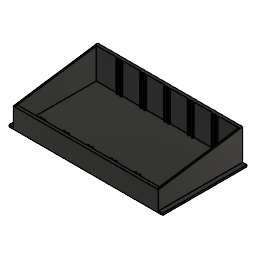
bin (Autodesk Fusion 360 design; units mm, degrees)
part number: 2026-08-18-20-33-51-830
Autodesk Fusion 360 part; units mm, degrees
sketch "Sketch1" plane through (0, 0, 0) normal (0, 0, 1) x (1, 0, 0)
  line L0 (-6, 0) -> (207, 0)
  line L1 (207, 0) -> (207, 117)
  line L2 (207, 117) -> (-6, 117)
  line L3 (-6, 117) -> (-6, 0)
extrude "Extrude1" add sketch "Sketch1" along normal blind 2.4 makes body 1
sketch "Sketch2" plane through (0, 0, 0) normal (0, 0, 1) x (1, 0, 0)
  line L0 (0, 0) -> (201, 0)
  line L1 (201, 0) -> (201, 4)
  line L2 (201, 4) -> (0, 4)
  line L3 (0, 4) -> (0, 0)
extrude "Extrude2" add sketch "Sketch2" along normal blind 28 separate body makes body 2
sketch "Sketch3" plane through (0, 0, 0) normal (0, 0, 1) x (1, 0, 0)
  line L0 (0, 113) -> (201, 113)
  line L1 (201, 113) -> (201, 117)
  line L2 (201, 117) -> (0, 117)
  line L3 (0, 117) -> (0, 113)
extrude "Extrude3" add sketch "Sketch3" along normal blind 45 separate body makes body 3
sketch "Sketch4" plane through (0, 0, 0) normal (1, 0, 0) x (0, 0, -1)
  line L0 (0, 0) -> (0, 117)
  line L1 (0, 117) -> (-45, 117)
  line L2 (-45, 117) -> (-28, 0)
  line L3 (-28, 0) -> (0, 0)
extrude "Extrude4" add sketch "Sketch4" along normal blind 2 separate body makes body 4
sketch "Sketch5" plane through (0, 0, 0) normal (1, 0, 0) x (0, 0, -1)
  line L0 (0, 0) -> (0, 117)
  line L1 (0, 117) -> (-45, 117)
  line L2 (-45, 117) -> (-28, 0)
  line L3 (-28, 0) -> (0, 0)
extrude "Extrude5" add sketch "Sketch5" along normal blind 2 from surface at 199 separate body makes body 5
sketch "Sketch6" plane through (0, 0, 0) normal (0, 0, 1) x (1, 0, 0)
  line L0 (31.4, 4) -> (33.4, 4)
  line L1 (33.4, 4) -> (33.4, 6)
  line L2 (33.4, 6) -> (31.4, 6)
  line L3 (31.4, 6) -> (31.4, 4)
extrude "Extrude6" add sketch "Sketch6" along normal blind 25.6 from surface at 2.4 separate body makes body 6
sketch "Sketch7" plane through (0, 0, 0) normal (0, 0, 1) x (1, 0, 0)
  line L0 (31.4, 111) -> (33.4, 111)
  line L1 (33.4, 111) -> (33.4, 113)
  line L2 (33.4, 113) -> (31.4, 113)
  line L3 (31.4, 113) -> (31.4, 111)
extrude "Extrude7" add sketch "Sketch7" along normal blind 42.6 from surface at 2.4 separate body makes body 7
sketch "Sketch8" plane through (0, 0, 0) normal (0, 0, 1) x (1, 0, 0)
  line L0 (36.6, 4) -> (38.6, 4)
  line L1 (38.6, 4) -> (38.6, 6)
  line L2 (38.6, 6) -> (36.6, 6)
  line L3 (36.6, 6) -> (36.6, 4)
extrude "Extrude8" add sketch "Sketch8" along normal blind 25.6 from surface at 2.4 separate body makes body 8
sketch "Sketch9" plane through (0, 0, 0) normal (0, 0, 1) x (1, 0, 0)
  line L0 (36.6, 111) -> (38.6, 111)
  line L1 (38.6, 111) -> (38.6, 113)
  line L2 (38.6, 113) -> (36.6, 113)
  line L3 (36.6, 113) -> (36.6, 111)
extrude "Extrude9" add sketch "Sketch9" along normal blind 42.6 from surface at 2.4 separate body makes body 9
sketch "Sketch10" plane through (0, 0, 0) normal (0, 0, 1) x (1, 0, 0)
  line L0 (64.4, 4) -> (66.4, 4)
  line L1 (66.4, 4) -> (66.4, 6)
  line L2 (66.4, 6) -> (64.4, 6)
  line L3 (64.4, 6) -> (64.4, 4)
extrude "Extrude10" add sketch "Sketch10" along normal blind 25.6 from surface at 2.4 separate body makes body 10
sketch "Sketch11" plane through (0, 0, 0) normal (0, 0, 1) x (1, 0, 0)
  line L0 (64.4, 111) -> (66.4, 111)
  line L1 (66.4, 111) -> (66.4, 113)
  line L2 (66.4, 113) -> (64.4, 113)
  line L3 (64.4, 113) -> (64.4, 111)
extrude "Extrude11" add sketch "Sketch11" along normal blind 42.6 from surface at 2.4 separate body makes body 11
sketch "Sketch12" plane through (0, 0, 0) normal (0, 0, 1) x (1, 0, 0)
  line L0 (69.6, 4) -> (71.6, 4)
  line L1 (71.6, 4) -> (71.6, 6)
  line L2 (71.6, 6) -> (69.6, 6)
  line L3 (69.6, 6) -> (69.6, 4)
extrude "Extrude12" add sketch "Sketch12" along normal blind 25.6 from surface at 2.4 separate body makes body 12
sketch "Sketch13" plane through (0, 0, 0) normal (0, 0, 1) x (1, 0, 0)
  line L0 (69.6, 111) -> (71.6, 111)
  line L1 (71.6, 111) -> (71.6, 113)
  line L2 (71.6, 113) -> (69.6, 113)
  line L3 (69.6, 113) -> (69.6, 111)
extrude "Extrude13" add sketch "Sketch13" along normal blind 42.6 from surface at 2.4 separate body makes body 13
sketch "Sketch14" plane through (0, 0, 0) normal (0, 0, 1) x (1, 0, 0)
  line L0 (97.4, 4) -> (99.4, 4)
  line L1 (99.4, 4) -> (99.4, 6)
  line L2 (99.4, 6) -> (97.4, 6)
  line L3 (97.4, 6) -> (97.4, 4)
extrude "Extrude14" add sketch "Sketch14" along normal blind 25.6 from surface at 2.4 separate body makes body 14
sketch "Sketch15" plane through (0, 0, 0) normal (0, 0, 1) x (1, 0, 0)
  line L0 (97.4, 111) -> (99.4, 111)
  line L1 (99.4, 111) -> (99.4, 113)
  line L2 (99.4, 113) -> (97.4, 113)
  line L3 (97.4, 113) -> (97.4, 111)
extrude "Extrude15" add sketch "Sketch15" along normal blind 42.6 from surface at 2.4 separate body makes body 15
sketch "Sketch16" plane through (0, 0, 0) normal (0, 0, 1) x (1, 0, 0)
  line L0 (102.6, 4) -> (104.6, 4)
  line L1 (104.6, 4) -> (104.6, 6)
  line L2 (104.6, 6) -> (102.6, 6)
  line L3 (102.6, 6) -> (102.6, 4)
extrude "Extrude16" add sketch "Sketch16" along normal blind 25.6 from surface at 2.4 separate body makes body 16
sketch "Sketch17" plane through (0, 0, 0) normal (0, 0, 1) x (1, 0, 0)
  line L0 (102.6, 111) -> (104.6, 111)
  line L1 (104.6, 111) -> (104.6, 113)
  line L2 (104.6, 113) -> (102.6, 113)
  line L3 (102.6, 113) -> (102.6, 111)
extrude "Extrude17" add sketch "Sketch17" along normal blind 42.6 from surface at 2.4 separate body makes body 17
sketch "Sketch18" plane through (0, 0, 0) normal (0, 0, 1) x (1, 0, 0)
  line L0 (130.4, 4) -> (132.4, 4)
  line L1 (132.4, 4) -> (132.4, 6)
  line L2 (132.4, 6) -> (130.4, 6)
  line L3 (130.4, 6) -> (130.4, 4)
extrude "Extrude18" add sketch "Sketch18" along normal blind 25.6 from surface at 2.4 separate body makes body 18
sketch "Sketch19" plane through (0, 0, 0) normal (0, 0, 1) x (1, 0, 0)
  line L0 (130.4, 111) -> (132.4, 111)
  line L1 (132.4, 111) -> (132.4, 113)
  line L2 (132.4, 113) -> (130.4, 113)
  line L3 (130.4, 113) -> (130.4, 111)
extrude "Extrude19" add sketch "Sketch19" along normal blind 42.6 from surface at 2.4 separate body makes body 19
sketch "Sketch20" plane through (0, 0, 0) normal (0, 0, 1) x (1, 0, 0)
  line L0 (135.6, 4) -> (137.6, 4)
  line L1 (137.6, 4) -> (137.6, 6)
  line L2 (137.6, 6) -> (135.6, 6)
  line L3 (135.6, 6) -> (135.6, 4)
extrude "Extrude20" add sketch "Sketch20" along normal blind 25.6 from surface at 2.4 separate body makes body 20
sketch "Sketch21" plane through (0, 0, 0) normal (0, 0, 1) x (1, 0, 0)
  line L0 (135.6, 111) -> (137.6, 111)
  line L1 (137.6, 111) -> (137.6, 113)
  line L2 (137.6, 113) -> (135.6, 113)
  line L3 (135.6, 113) -> (135.6, 111)
extrude "Extrude21" add sketch "Sketch21" along normal blind 42.6 from surface at 2.4 separate body makes body 21
sketch "Sketch22" plane through (0, 0, 0) normal (0, 0, 1) x (1, 0, 0)
  line L0 (163.4, 4) -> (165.4, 4)
  line L1 (165.4, 4) -> (165.4, 6)
  line L2 (165.4, 6) -> (163.4, 6)
  line L3 (163.4, 6) -> (163.4, 4)
extrude "Extrude22" add sketch "Sketch22" along normal blind 25.6 from surface at 2.4 separate body makes body 22
sketch "Sketch23" plane through (0, 0, 0) normal (0, 0, 1) x (1, 0, 0)
  line L0 (163.4, 111) -> (165.4, 111)
  line L1 (165.4, 111) -> (165.4, 113)
  line L2 (165.4, 113) -> (163.4, 113)
  line L3 (163.4, 113) -> (163.4, 111)
extrude "Extrude23" add sketch "Sketch23" along normal blind 42.6 from surface at 2.4 separate body makes body 23
sketch "Sketch24" plane through (0, 0, 0) normal (0, 0, 1) x (1, 0, 0)
  line L0 (168.6, 4) -> (170.6, 4)
  line L1 (170.6, 4) -> (170.6, 6)
  line L2 (170.6, 6) -> (168.6, 6)
  line L3 (168.6, 6) -> (168.6, 4)
extrude "Extrude24" add sketch "Sketch24" along normal blind 25.6 from surface at 2.4 separate body makes body 24
sketch "Sketch25" plane through (0, 0, 0) normal (0, 0, 1) x (1, 0, 0)
  line L0 (168.6, 111) -> (170.6, 111)
  line L1 (170.6, 111) -> (170.6, 113)
  line L2 (170.6, 113) -> (168.6, 113)
  line L3 (168.6, 113) -> (168.6, 111)
extrude "Extrude25" add sketch "Sketch25" along normal blind 42.6 from surface at 2.4 separate body makes body 25
combine "Combine1" operation add target body 1 tool bodies 2 3 4 5 6 7 8 9 10 11 12 13 14 15 16 17 18 19 20 21 22 23 24 25
named bodies: "Тело"
